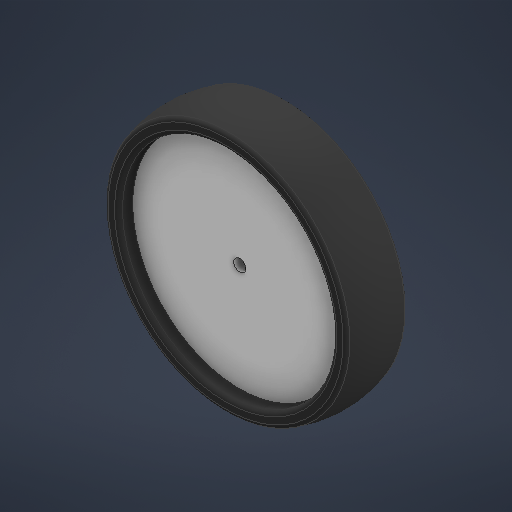
# Autodesk Inventor part: drive and dribbler wheel
Saved by Autodesk Inventor 2026.1 (Build 301233000, 233)
## iProperties
Created: 2024-09-20
Part Number: drive and dribbler wheel
Material: Generisch
Document SubType Name: Modeling
Designer: Familie Steib
Density: 1 g/cm^3
Appearance: Vorgabe
Author: Familie Steib
Autodesk Inventor part; units mm, degrees
ref_plane "YZ Plane" through (0, 0, 0) normal (1, 0, 0) x (0, 1, 0)
ref_plane "XZ Plane" through (0, 0, 0) normal (0, 1, 0) x (-1, 0, 0)
ref_plane "XY Plane" through (0, 0, 0) normal (0, 0, 1) x (1, 0, 0)
sketch "Skizze1" plane through (0, 0, 0) normal (0, 0, 1) x (1, 0, 0)
  circle A0 centre (0, 0) radius 26.5
  circle A1 centre (0, 0) radius 32.5
  circle A2 centre (0, 0) radius 5
  circle A3 centre (0, 0) radius 1.5
  dimension "d0" = 53
  dimension "d1" = 65
  dimension "d2" = 10
  dimension "d3" = 3
  constraints: 4 centre point, 4 coincident
  measures "d0" diameter of A0
  measures "d1" diameter of A1
  measures "d2" diameter of A2
  measures "d3" diameter of A3
extrude "Extrusion1" add sketch "Skizze1" along normal mid plane 15 contours A1
extrude "Extrusion2" add sketch "Skizze1" along normal mid plane 8 contours A0 | A2
chamfer "Fase2" distance 7.5 angle 20 2 edges at (-32.5, 0, -7.5) (-32.5, 0, 7.5) measured on face at (-32.5, 0, -7) measured on face at (-32.5, 0, 7)
fillet "Rundung2" radius 22 3 edges at (-32.5, 0, 0.0001) (-32.5, 0, 0) (-32.5, 0, -0.0001)
fillet "Rundung3" radius 1 4 edges at (-29.7703, -0.0011, -7.5) (-26.5, 0, -7.5) (-29.7703, -0.0011, 7.5) (-26.5, 0, 7.5)
